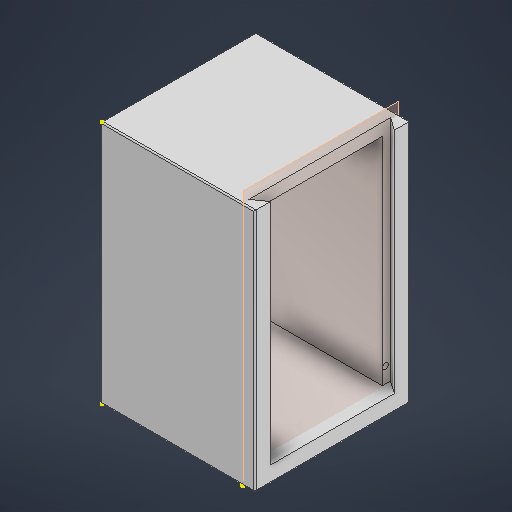
# Autodesk Inventor part: Part4
Saved by Autodesk Inventor 2026.1 (Build 301233000, 233)
## iProperties
Created: 2025-08-22
Part Number: Part4
Material: Generic
Document SubType Name: Modeling
Designer: usman
Density: 1 g/cm^3
Appearance: Default
Author: usman
Autodesk Inventor part; units mm, degrees
(part 1 of 2)
ref_plane "YZ Plane" through (0, 0, 0) normal (1, 0, 0) x (0, 1, 0)
ref_plane "XZ Plane" through (0, 0, 0) normal (0, 1, 0) x (-1, 0, 0)
ref_plane "XY Plane" through (0, 0, 0) normal (0, 0, 1) x (1, 0, 0)
sketch "Sketch1" plane through (0, 0, 0) normal (1, 0, 0) x (0, 1, 0)
  line L0 (0, 0) -> (191.4, 0)
  line L1 (191.4, 0) -> (191.4, -121.8)
  line L2 (191.4, -121.8) -> (0, -121.8)
  line L3 (0, -121.8) -> (0, 0)
  dimension "d0" = 191.4
  dimension "d1" = 121.8
  constraints: 8 end point, 2 parallel, 1 horizontal, 1 perpendicular
  measures "d0" distance of L0.start L0.end
  measures "d1" distance of L0.end L1.end
extrude "Extrusion1" add sketch "Sketch1" along normal blind 120
sketch "Sketch2" plane through (120, 0, 0) normal (1, 0, 0) x (0, 0, -1)
  line L0 (12.4, 178.9) -> (109.4, 178.9)
  line L1 (109.4, 178.9) -> (109.4, 12.5)
  line L2 (109.4, 12.5) -> (12.4, 12.5)
  line L3 (12.4, 12.5) -> (12.4, 178.9)
  line L4 (121.8, 191.4) -> (0, 191.4) projected
  line L5 (0, 0) -> (121.8, 0) projected
  line L6 (0, 191.4) -> (0, 0) projected
  dimension "d4" = 12.5
  dimension "d5" = 12.5
  dimension "d6" = 12.4
  dimension "d7" = 97
  constraints: 8 end point, 2 parallel, 1 horizontal, 1 perpendicular
  measures "d4" distance between parallel lines of L4 L0
  measures "d5" distance between parallel lines of L5 L2
  measures "d6" distance between parallel lines of L6 L3
  measures "d7" distance of L1.end L2.end
extrude "Extrusion2" cut sketch "Sketch2" against normal blind 105
sketch "Sketch3" plane through (0, 191.4, 0) normal (0, 1, 0) x (1, 0, 0)
  point P0 (0, 0)
sketch "Sketch4" plane through (0, 191.4, 0) normal (0, 1, 0) x (1, 0, 0)
  line L0 (120, 109.4) -> (15, 109.4) projected
  line L1 (120, 109.4) -> (110, 116.4021)
  line L2 (120, 121.8) -> (120, 0) projected
  line L3 (120, 60.9) -> (110, 60.9)
  line L4 (110, 60.9) -> (110, 116.4021)
  line L5 (120, 109.4) -> (120, 60.9)
  point P0 (0, 0)
  point P1 (106.1473, 60.9)
  dimension "d10" = 55
  dimension "d11" = 10
  constraints: 8 end point, 1 collinear, 1 horizontal, 1 midpoint, 1 perpendicular
  measures "d10" angle of L2 L1
  measures "d11" horizontal distance of L0.start L1.end
extrude "Extrusion3" cut sketch "Sketch4" against normal up to surface (178.9 mm away)
sketch "Sketch5" plane through (0, 191.4, 0) normal (0, 1, 0) x (1, 0, 0)
  line L0 (120, 109.4) -> (120, 12.4) projected
  line L1 (120, 12.4) -> (15, 12.4) projected
  line L2 (120, 60.9) -> (120, 12.4)
  line L3 (120, 12.4) -> (110, 5.3979)
  line L4 (120, 60.9) -> (120, 0) projected
  line L5 (110, 109.4) -> (110, 60.9) projected
  line L6 (110, 60.9) -> (110, 5.3979)
  line L7 (110, 60.9) -> (110, 5.3979)
  line L8 (110, 60.9) -> (120, 60.9) projected
  line L9 (120, 60.9) -> (110, 60.9)
  point P0 (0, 0)
  dimension "d14" = 10
  dimension "d15" = 125
  constraints: 10 end point, 2 collinear, 1 midpoint, 1 perpendicular, 1 vertical
  measures "d14" horizontal distance of L0.end L3.end
  measures "d15" angle of L4 L3
extrude "Extrusion4" cut sketch "Sketch5" against normal up to surface (178.9 mm away)
fillet "Fillet1" radius 1 7 edges at (60, 191.4, 0) (60, 0, 0) (60, 191.4, -121.8) (60, 0, -121.8) (120, 95.7, -121.8) (120, 0, -60.9) (120, 95.7, 0)
sketch "Sketch7" plane through (0, 0, -120.8) normal (0, -1, 0) x (1, 0, 0)
  point P0 (0, 120.8)
sketch "Sketch9" plane through (0, 0, -120.8) normal (0, -1, 0) x (1, 0, 0)
  line L0 (38.885, 112.5851) -> (86.602, 112.5851) construction
  line L1 (86.602, 112.5851) -> (86.602, 8.2699) construction
  line L2 (86.602, 8.2699) -> (38.885, 8.2699) construction
  line L3 (38.885, 8.2699) -> (38.885, 112.5851) construction
  line L4 (41.713, 65.0369) -> (41.7857, 63.9578)
  line L5 (41.7857, 63.9578) -> (41.713, 63.9578)
  spline S0 degree 2 poles (41.713, 63.9578) (41.5678, 64.4429) (41.0308, 64.8709) (40.6547, 64.8709) knots 0 0 0 1 2 2 2
  spline S1 degree 2 poles (40.6547, 64.8709) (40.3408, 64.8709) (39.8324, 64.5492) (39.5393, 63.8463) (39.5393, 63.3223) knots 0 0 0 1 2 3 3 3
  spline S2 degree 2 poles (39.5393, 63.3223) (39.5393, 62.8917) (39.8143, 62.2588) (40.3694, 61.9216) (40.7221, 61.9216) knots 0 0 0 1 2 3 3 3
  spline S3 degree 2 poles (40.7221, 61.9216) (41.0308, 61.9216) (41.5029, 62.1861) (41.7857, 62.5804) knots 0 0 0 1 2 2 2
  line L6 (41.7857, 62.5804) -> (41.8583, 62.5337)
  spline S4 degree 2 poles (41.8583, 62.5337) (41.6196, 62.1109) (40.9841, 61.7166) (40.5457, 61.7166) knots 0 0 0 1 2 2 2
  spline S5 degree 2 poles (40.5457, 61.7166) (39.7572, 61.7166) (39.324, 62.3029) knots 0 0 0 1 1 1
  spline S6 degree 2 poles (39.324, 62.3029) (39.0023, 62.7387) (39.0023, 63.3275) knots 0 0 0 1 1 1
  spline S7 degree 2 poles (39.0023, 63.3275) (39.0023, 63.8022) (39.4278, 64.5985) (40.1748, 65.0369) (40.6158, 65.0369) knots 0 0 0 1 2 3 3 3
  spline S8 degree 2 poles (40.6158, 65.0369) (40.9582, 65.0369) (41.2928, 64.8683) knots 0 0 0 1 1 1
  spline S9 degree 2 poles (41.2928, 64.8683) (41.3914, 64.8164) (41.4329, 64.8164) knots 0 0 0 1 1 1
  spline S10 degree 2 poles (41.4329, 64.8164) (41.4977, 64.8164) (41.5444, 64.8605) knots 0 0 0 1 1 1
  spline S11 degree 2 poles (41.5444, 64.8605) (41.6041, 64.9254) (41.63, 65.0369) knots 0 0 0 1 1 1
  line L7 (41.63, 65.0369) -> (41.713, 65.0369)
  spline S12 degree 2 poles (43.3887, 62.1005) (43.0593, 61.8437) (42.9737, 61.8048) knots 0 0 0 1 1 1
  spline S13 degree 2 poles (42.9737, 61.8048) (42.8492, 61.7452) (42.7065, 61.7452) knots 0 0 0 1 1 1
  spline S14 degree 2 poles (42.7065, 61.7452) (42.4834, 61.7452) (42.1955, 62.0487) (42.1955, 62.2977) knots 0 0 0 1 2 2 2
  spline S15 degree 2 poles (42.1955, 62.2977) (42.1955, 62.4533) (42.2655, 62.5701) knots 0 0 0 1 1 1
  spline S16 degree 2 poles (42.2655, 62.5701) (42.3615, 62.7283) (42.8362, 63.0084) (43.3887, 63.2108) knots 0 0 0 1 2 2 2
  line L8 (43.3887, 63.2108) -> (43.3887, 63.2938)
  spline S17 degree 2 poles (43.3887, 63.2938) (43.3887, 63.6154) (43.1864, 63.8541) (42.9918, 63.8541) knots 0 0 0 1 2 2 2
  spline S18 degree 2 poles (42.9918, 63.8541) (42.8466, 63.8541) (42.7584, 63.7736) knots 0 0 0 1 1 1
  spline S19 degree 2 poles (42.7584, 63.7736) (42.6702, 63.6958) (42.6702, 63.5921) knots 0 0 0 1 1 1
  line L9 (42.6702, 63.5921) -> (42.6754, 63.4572)
  spline S20 degree 2 poles (42.6754, 63.4572) (42.6754, 63.3482) (42.5638, 63.2315) (42.4757, 63.2315) knots 0 0 0 1 2 2 2
  spline S21 degree 2 poles (42.4757, 63.2315) (42.39, 63.2315) (42.2785, 63.3534) (42.2785, 63.4598) knots 0 0 0 1 2 2 2
  spline S22 degree 2 poles (42.2785, 63.4598) (42.2785, 63.6595) (42.6909, 63.9967) (43.0619, 63.9967) knots 0 0 0 1 2 2 2
  spline S23 degree 2 poles (43.0619, 63.9967) (43.3472, 63.9967) (43.5288, 63.9008) knots 0 0 0 1 1 1
  spline S24 degree 2 poles (43.5288, 63.9008) (43.6689, 63.8281) (43.7337, 63.6751) knots 0 0 0 1 1 1
  spline S25 degree 2 poles (43.7337, 63.6751) (43.7752, 63.5739) (43.7752, 63.2626) knots 0 0 0 1 1 1
  line L10 (43.7752, 63.2626) -> (43.7752, 62.5337)
  spline S26 degree 2 poles (43.7752, 62.5337) (43.7752, 62.2277) (43.7986, 62.0902) (43.853, 62.0435) (43.8868, 62.0435) knots 0 0 0 1 2 3 3 3
  spline S27 degree 2 poles (43.8868, 62.0435) (43.9257, 62.0435) (43.9542, 62.059) knots 0 0 0 1 1 1
  spline S28 degree 2 poles (43.9542, 62.059) (44.0035, 62.0902) (44.1436, 62.2302) knots 0 0 0 1 1 1
  line L11 (44.1436, 62.2302) -> (44.1436, 62.1005)
  spline S29 degree 2 poles (44.1436, 62.1005) (43.8816, 61.7478) (43.6429, 61.7478) knots 0 0 0 1 1 1
  spline S30 degree 2 poles (43.6429, 61.7478) (43.5262, 61.7478) (43.3913, 61.906) (43.3887, 62.1005) knots 0 0 0 1 2 2 2
  line L12 (43.3887, 62.251) -> (43.3887, 63.0681)
  spline S31 degree 2 poles (43.3887, 63.0681) (43.0359, 62.928) (42.9322, 62.8684) knots 0 0 0 1 1 1
  spline S32 degree 2 poles (42.9322, 62.8684) (42.748, 62.7672) (42.5898, 62.5415) (42.5898, 62.4092) knots 0 0 0 1 2 2 2
  spline S33 degree 2 poles (42.5898, 62.4092) (42.5898, 62.2406) (42.7895, 62.0175) (42.9218, 62.0175) knots 0 0 0 1 2 2 2
  spline S34 degree 2 poles (42.9218, 62.0175) (43.0982, 62.0175) (43.3887, 62.251) knots 0 0 0 1 1 1
  line L13 (45.6896, 63.9967) -> (45.6896, 63.2652)
  line L14 (45.6896, 63.2652) -> (45.6117, 63.2652)
  spline S35 degree 2 poles (45.6117, 63.2652) (45.5235, 63.6102) (45.246, 63.8592) (45.0307, 63.8592) knots 0 0 0 1 2 2 2
  spline S36 degree 2 poles (45.0307, 63.8592) (44.8673, 63.8592) (44.6649, 63.6855) (44.6649, 63.5817) knots 0 0 0 1 2 2 2
  spline S37 degree 2 poles (44.6649, 63.5817) (44.6649, 63.4494) (44.7402, 63.356) knots 0 0 0 1 1 1
  spline S38 degree 2 poles (44.7402, 63.356) (44.8102, 63.26) (45.0333, 63.1511) knots 0 0 0 1 1 1
  line L15 (45.0333, 63.1511) -> (45.3757, 62.9851)
  spline S39 degree 2 poles (45.3757, 62.9851) (45.8504, 62.7542) (45.8504, 62.3755) knots 0 0 0 1 1 1
  spline S40 degree 2 poles (45.8504, 62.3755) (45.8504, 62.0824) (45.4094, 61.7244) (45.1345, 61.7244) knots 0 0 0 1 2 2 2
  spline S41 degree 2 poles (45.1345, 61.7244) (44.9373, 61.7244) (44.6857, 61.7945) knots 0 0 0 1 1 1
  spline S42 degree 2 poles (44.6857, 61.7945) (44.6079, 61.8178) (44.5586, 61.8178) knots 0 0 0 1 1 1
  spline S43 degree 2 poles (44.5586, 61.8178) (44.5067, 61.8178) (44.4756, 61.7581) knots 0 0 0 1 1 1
  line L16 (44.4756, 61.7581) -> (44.3978, 61.7581)
  line L17 (44.3978, 61.7581) -> (44.3978, 62.5234)
  line L18 (44.3978, 62.5234) -> (44.4756, 62.5234)
  spline S44 degree 2 poles (44.4756, 62.5234) (44.5404, 62.1939) (44.9088, 61.8619) (45.1396, 61.8619) knots 0 0 0 1 2 2 2
  spline S45 degree 2 poles (45.1396, 61.8619) (45.3005, 61.8619) (45.5028, 62.0513) (45.5028, 62.1861) knots 0 0 0 1 2 2 2
  spline S46 degree 2 poles (45.5028, 62.1861) (45.5028, 62.347) (45.2771, 62.5675) (44.5975, 62.9021) (44.4912, 63.0396) knots 0 0 0 1 2 3 3 3
  spline S47 degree 2 poles (44.4912, 63.0396) (44.3874, 63.1718) (44.3874, 63.3768) knots 0 0 0 1 1 1
  spline S48 degree 2 poles (44.3874, 63.3768) (44.3874, 63.6414) (44.7505, 63.9967) (45.0385, 63.9967) knots 0 0 0 1 2 2 2
  spline S49 degree 2 poles (45.0385, 63.9967) (45.1656, 63.9967) (45.3446, 63.9423) knots 0 0 0 1 1 1
  spline S50 degree 2 poles (45.3446, 63.9423) (45.4639, 63.9085) (45.5028, 63.9085) knots 0 0 0 1 1 1
  spline S51 degree 2 poles (45.5028, 63.9085) (45.5417, 63.9085) (45.5832, 63.9423) (45.6117, 63.9967) knots 0 0 0 1 2 2 2
  line L19 (45.6117, 63.9967) -> (45.6896, 63.9967)
  line L20 (46.9113, 63.9967) -> (46.9113, 62.2743)
  spline S52 degree 2 poles (46.9113, 62.2743) (46.9113, 62.0746) (46.9684, 61.9397) (47.0851, 61.8749) (47.2356, 61.8749) knots 0 0 0 1 2 3 3 3
  line L21 (47.2356, 61.8749) -> (47.2356, 61.7893)
  line L22 (47.2356, 61.7893) -> (46.1954, 61.7893)
  line L23 (46.1954, 61.7893) -> (46.1954, 61.8749)
  spline S53 degree 2 poles (46.1954, 61.8749) (46.351, 61.8749) (46.46, 61.9345) (46.5222, 62.0746) (46.5222, 62.2743) knots 0 0 0 1 2 3 3 3
  line L24 (46.5222, 62.2743) -> (46.5222, 63.0992)
  spline S54 degree 2 poles (46.5222, 63.0992) (46.5222, 63.4468) (46.5015, 63.5506) knots 0 0 0 1 1 1
  spline S55 degree 2 poles (46.5015, 63.5506) (46.4859, 63.6258) (46.4133, 63.6855) (46.3536, 63.6855) knots 0 0 0 1 2 2 2
  spline S56 degree 2 poles (46.3536, 63.6855) (46.2888, 63.6855) (46.1954, 63.6491) knots 0 0 0 1 1 1
  line L25 (46.1954, 63.6491) -> (46.1617, 63.7347)
  line L26 (46.1617, 63.7347) -> (46.8076, 63.9967)
  line L27 (46.8076, 63.9967) -> (46.9113, 63.9967)
  spline S57 degree 2 poles (46.7168, 65.1199) (46.8153, 65.1199) (46.9528, 64.9824) (46.9528, 64.8839) knots 0 0 0 1 2 2 2
  spline S58 degree 2 poles (46.9528, 64.8839) (46.9528, 64.7853) (46.8153, 64.6452) (46.7168, 64.6452) knots 0 0 0 1 2 2 2
  spline S59 degree 2 poles (46.7168, 64.6452) (46.6182, 64.6452) (46.4781, 64.7853) (46.4781, 64.8839) knots 0 0 0 1 2 2 2
  spline S60 degree 2 poles (46.4781, 64.8839) (46.4781, 64.9824) (46.6156, 65.1199) (46.7168, 65.1199) knots 0 0 0 1 2 2 2
  spline S61 degree 2 poles (48.1331, 63.5428) (48.5092, 63.9967) (48.8516, 63.9967) knots 0 0 0 1 1 1
  spline S62 degree 2 poles (48.8516, 63.9967) (49.0254, 63.9967) (49.277, 63.8203) (49.3522, 63.6206) knots 0 0 0 1 2 2 2
  spline S63 degree 2 poles (49.3522, 63.6206) (49.4041, 63.4805) (49.4041, 63.19) knots 0 0 0 1 1 1
  line L28 (49.4041, 63.19) -> (49.4041, 62.2743)
  spline S64 degree 2 poles (49.4041, 62.2743) (49.4041, 62.072) (49.4378, 61.9994) knots 0 0 0 1 1 1
  spline S65 degree 2 poles (49.4378, 61.9994) (49.4638, 61.9397) (49.5779, 61.8749) (49.7309, 61.8749) knots 0 0 0 1 2 2 2
  line L29 (49.7309, 61.8749) -> (49.7309, 61.7893)
  line L30 (49.7309, 61.7893) -> (48.6674, 61.7893)
  line L31 (48.6674, 61.7893) -> (48.6674, 61.8749)
  line L32 (48.6674, 61.8749) -> (48.7115, 61.8749)
  spline S66 degree 2 poles (48.7115, 61.8749) (48.862, 61.8749) (48.9813, 61.9657) (49.0046, 62.0539) knots 0 0 0 1 2 2 2
  spline S67 degree 2 poles (49.0046, 62.0539) (49.015, 62.0902) (49.015, 62.2743) knots 0 0 0 1 1 1
  line L33 (49.015, 62.2743) -> (49.015, 63.1511)
  spline S68 degree 2 poles (49.015, 63.1511) (49.015, 63.4442) (48.8646, 63.7088) (48.6856, 63.7088) knots 0 0 0 1 2 2 2
  spline S69 degree 2 poles (48.6856, 63.7088) (48.408, 63.7088) (48.1331, 63.4053) knots 0 0 0 1 1 1
  line L34 (48.1331, 63.4053) -> (48.1331, 62.2743)
  spline S70 degree 2 poles (48.1331, 62.2743) (48.1331, 62.0564) (48.159, 62.0046) knots 0 0 0 1 1 1
  spline S71 degree 2 poles (48.159, 62.0046) (48.1927, 61.9371) (48.3069, 61.8749) (48.4832, 61.8749) knots 0 0 0 1 2 2 2
  line L35 (48.4832, 61.8749) -> (48.4832, 61.7893)
  line L36 (48.4832, 61.7893) -> (47.4171, 61.7893)
  line L37 (47.4171, 61.7893) -> (47.4171, 61.8749)
  line L38 (47.4171, 61.8749) -> (47.4638, 61.8749)
  spline S72 degree 2 poles (47.4638, 61.8749) (47.6298, 61.8749) (47.744, 62.0409) (47.744, 62.2743) knots 0 0 0 1 2 2 2
  line L39 (47.744, 62.2743) -> (47.744, 63.0707)
  spline S73 degree 2 poles (47.744, 63.0707) (47.744, 63.4546) (47.7077, 63.6232) (47.635, 63.6855) (47.5754, 63.6855) knots 0 0 0 1 2 3 3 3
  spline S74 degree 2 poles (47.5754, 63.6855) (47.5105, 63.6855) (47.4197, 63.6491) knots 0 0 0 1 1 1
  line L40 (47.4197, 63.6491) -> (47.3834, 63.7347)
  line L41 (47.3834, 63.7347) -> (48.0319, 63.9967)
  line L42 (48.0319, 63.9967) -> (48.1331, 63.9967)
  line L43 (48.1331, 63.9967) -> (48.1331, 63.5428)
  spline S75 degree 2 poles (50.478, 62.5726) (50.2809, 62.6686) (50.0707, 63.011) (50.0707, 63.2211) knots 0 0 0 1 2 2 2
  spline S76 degree 2 poles (50.0707, 63.2211) (50.0707, 63.5376) (50.5506, 63.9967) (50.9268, 63.9967) knots 0 0 0 1 2 2 2
  spline S77 degree 2 poles (50.9268, 63.9967) (51.2328, 63.9967) (51.4585, 63.8463) knots 0 0 0 1 1 1
  line L44 (51.4585, 63.8463) -> (51.9125, 63.8463)
  spline S78 degree 2 poles (51.9125, 63.8463) (52.0136, 63.8463) (52.0473, 63.8359) (52.0551, 63.8203) knots 0 0 0 1 2 2 2
  spline S79 degree 2 poles (52.0551, 63.8203) (52.0681, 63.7996) (52.0681, 63.7451) knots 0 0 0 1 1 1
  spline S80 degree 2 poles (52.0681, 63.7451) (52.0681, 63.6855) (52.0551, 63.6621) knots 0 0 0 1 1 1
  spline S81 degree 2 poles (52.0551, 63.6621) (52.0499, 63.6491) (52.0136, 63.6362) (51.9125, 63.6362) knots 0 0 0 1 2 2 2
  line L45 (51.9125, 63.6362) -> (51.6323, 63.6362)
  spline S82 degree 2 poles (51.6323, 63.6362) (51.7646, 63.4676) (51.7646, 63.2056) knots 0 0 0 1 1 1
  spline S83 degree 2 poles (51.7646, 63.2056) (51.7646, 62.9047) (51.3055, 62.4793) (50.919, 62.4793) knots 0 0 0 1 2 2 2
  spline S84 degree 2 poles (50.919, 62.4793) (50.7607, 62.4793) (50.5921, 62.526) knots 0 0 0 1 1 1
  spline S85 degree 2 poles (50.5921, 62.526) (50.491, 62.4378) (50.4183, 62.3055) (50.4183, 62.2588) knots 0 0 0 1 2 2 2
  spline S86 degree 2 poles (50.4183, 62.2588) (50.4183, 62.2173) (50.4962, 62.142) (50.6077, 62.1265) knots 0 0 0 1 2 2 2
  spline S87 degree 2 poles (50.6077, 62.1265) (50.6725, 62.1161) (50.9371, 62.1109) knots 0 0 0 1 1 1
  spline S88 degree 2 poles (50.9371, 62.1109) (51.4196, 62.098) (51.5623, 62.0772) knots 0 0 0 1 1 1
  spline S89 degree 2 poles (51.5623, 62.0772) (51.7802, 62.0461) (52.0396, 61.7841) (52.0396, 61.5947) knots 0 0 0 1 2 2 2
  spline S90 degree 2 poles (52.0396, 61.5947) (52.0396, 61.3301) (51.7905, 61.0993) knots 0 0 0 1 1 1
  spline S91 degree 2 poles (51.7905, 61.0993) (51.4248, 60.7569) (50.836, 60.7569) knots 0 0 0 1 1 1
  spline S92 degree 2 poles (50.836, 60.7569) (50.3846, 60.7569) (50.0733, 60.9592) knots 0 0 0 1 1 1
  spline S93 degree 2 poles (50.0733, 60.9592) (49.897, 61.0759) (49.897, 61.203) knots 0 0 0 1 1 1
  spline S94 degree 2 poles (49.897, 61.203) (49.897, 61.2601) (49.9229, 61.3146) knots 0 0 0 1 1 1
  spline S95 degree 2 poles (49.9229, 61.3146) (49.9618, 61.4028) (50.0863, 61.5558) knots 0 0 0 1 1 1
  spline S96 degree 2 poles (50.0863, 61.5558) (50.1045, 61.5766) (50.325, 61.8074) knots 0 0 0 1 1 1
  spline S97 degree 2 poles (50.325, 61.8074) (50.2056, 61.8801) (50.1045, 61.9968) (50.1045, 62.0694) knots 0 0 0 1 2 2 2
  spline S98 degree 2 poles (50.1045, 62.0694) (50.1045, 62.1498) (50.2368, 62.3703) (50.478, 62.5726) knots 0 0 0 1 2 2 2
  spline S99 degree 2 poles (50.4547, 61.7893) (50.3431, 61.67) (50.2316, 61.465) (50.2316, 61.3794) knots 0 0 0 1 2 2 2
  spline S100 degree 2 poles (50.2316, 61.3794) (50.2316, 61.2679) (50.3665, 61.1849) knots 0 0 0 1 1 1
  spline S101 degree 2 poles (50.3665, 61.1849) (50.6025, 61.0396) (51.0461, 61.0396) knots 0 0 0 1 1 1
  spline S102 degree 2 poles (51.0461, 61.0396) (51.4663, 61.0396) (51.8684, 61.3353) (51.8684, 61.5013) knots 0 0 0 1 2 2 2
  spline S103 degree 2 poles (51.8684, 61.5013) (51.8684, 61.6233) (51.749, 61.6751) knots 0 0 0 1 1 1
  spline S104 degree 2 poles (51.749, 61.6751) (51.6271, 61.7244) (51.2666, 61.7348) knots 0 0 0 1 1 1
  spline S105 degree 2 poles (51.2666, 61.7348) (50.7374, 61.7478) (50.4547, 61.7893) knots 0 0 0 1 1 1
  spline S106 degree 2 poles (50.8852, 63.8852) (50.7115, 63.8852) (50.478, 63.6102) (50.478, 63.3249) knots 0 0 0 1 2 2 2
  spline S107 degree 2 poles (50.478, 63.3249) (50.478, 62.954) (50.6362, 62.7516) knots 0 0 0 1 1 1
  spline S108 degree 2 poles (50.6362, 62.7516) (50.7581, 62.596) (50.9475, 62.596) knots 0 0 0 1 1 1
  spline S109 degree 2 poles (50.9475, 62.596) (51.1239, 62.596) (51.3548, 62.8632) (51.3548, 63.1485) knots 0 0 0 1 2 2 2
  spline S110 degree 2 poles (51.3548, 63.1485) (51.3548, 63.5194) (51.1939, 63.7295) knots 0 0 0 1 1 1
  spline S111 degree 2 poles (51.1939, 63.7295) (51.0746, 63.8852) (50.8852, 63.8852) knots 0 0 0 1 1 1
  line L46 (54.343, 63.7659) -> (54.343, 62.3548)
  spline S112 degree 2 poles (54.343, 62.3548) (54.343, 62.0564) (54.4078, 61.9786) knots 0 0 0 1 1 1
  spline S113 degree 2 poles (54.4078, 61.9786) (54.496, 61.8749) (54.6413, 61.8749) knots 0 0 0 1 1 1
  line L47 (54.6413, 61.8749) -> (54.8358, 61.8749)
  line L48 (54.8358, 61.8749) -> (54.8358, 61.7893)
  line L49 (54.8358, 61.7893) -> (53.5518, 61.7893)
  line L50 (53.5518, 61.7893) -> (53.5518, 61.8749)
  line L51 (53.5518, 61.8749) -> (53.6478, 61.8749)
  spline S114 degree 2 poles (53.6478, 61.8749) (53.7412, 61.8749) (53.8942, 61.9683) (53.9539, 62.1265) (53.9539, 62.3548) knots 0 0 0 1 2 3 3 3
  line L52 (53.9539, 62.3548) -> (53.9539, 63.7659)
  line L53 (53.9539, 63.7659) -> (53.5363, 63.7659)
  line L54 (53.5363, 63.7659) -> (53.5363, 63.9345)
  line L55 (53.5363, 63.9345) -> (53.9539, 63.9345)
  line L56 (53.9539, 63.9345) -> (53.9539, 64.0745)
  spline S115 degree 2 poles (53.9539, 64.0745) (53.9539, 64.3962) (54.1614, 64.8398) (54.5868, 65.1147) (54.8514, 65.1147) knots 0 0 0 1 2 3 3 3
  spline S116 degree 2 poles (54.8514, 65.1147) (55.0978, 65.1147) (55.3053, 64.9565) knots 0 0 0 1 1 1
  spline S117 degree 2 poles (55.3053, 64.9565) (55.4402, 64.8501) (55.4402, 64.7204) knots 0 0 0 1 1 1
  spline S118 degree 2 poles (55.4402, 64.7204) (55.4402, 64.6504) (55.3183, 64.5259) (55.2483, 64.5259) knots 0 0 0 1 2 2 2
  spline S119 degree 2 poles (55.2483, 64.5259) (55.1938, 64.5259) (55.0745, 64.6037) (54.9007, 64.8579) (54.8281, 64.902) knots 0 0 0 1 2 3 3 3
  spline S120 degree 2 poles (54.8281, 64.902) (54.7554, 64.9461) (54.6672, 64.9461) knots 0 0 0 1 1 1
  spline S121 degree 2 poles (54.6672, 64.9461) (54.5583, 64.9461) (54.4078, 64.832) (54.343, 64.5907) (54.343, 64.0901) knots 0 0 0 1 2 3 3 3
  line L57 (54.343, 64.0901) -> (54.343, 63.9345)
  line L58 (54.343, 63.9345) -> (54.8955, 63.9345)
  line L59 (54.8955, 63.9345) -> (54.8955, 63.7659)
  line L60 (54.8955, 63.7659) -> (54.343, 63.7659)
  spline S122 degree 2 poles (56.1484, 63.9967) (56.636, 63.9967) (56.9292, 63.6258) knots 0 0 0 1 1 1
  spline S123 degree 2 poles (56.9292, 63.6258) (57.1808, 63.3119) (57.1808, 62.9021) knots 0 0 0 1 1 1
  spline S124 degree 2 poles (57.1808, 62.9021) (57.1808, 62.6141) (56.9032, 62.0227) (56.4207, 61.7244) (56.1224, 61.7244) knots 0 0 0 1 2 3 3 3
  spline S125 degree 2 poles (56.1224, 61.7244) (55.6374, 61.7244) (55.352, 62.1109) knots 0 0 0 1 1 1
  spline S126 degree 2 poles (55.352, 62.1109) (55.1108, 62.4352) (55.1108, 62.8398) knots 0 0 0 1 1 1
  spline S127 degree 2 poles (55.1108, 62.8398) (55.1108, 63.1355) (55.4039, 63.7192) (55.8812, 63.9967) (56.1484, 63.9967) knots 0 0 0 1 2 3 3 3
  spline S128 degree 2 poles (56.0758, 63.8437) (55.9512, 63.8437) (55.7022, 63.6958) (55.5466, 63.3275) (55.5466, 63.037) knots 0 0 0 1 2 3 3 3
  spline S129 degree 2 poles (55.5466, 63.037) (55.5466, 62.5701) (55.9175, 61.8904) (56.2236, 61.8904) knots 0 0 0 1 2 2 2
  spline S130 degree 2 poles (56.2236, 61.8904) (56.4493, 61.8904) (56.745, 62.264) (56.745, 62.7205) knots 0 0 0 1 2 2 2
  spline S131 degree 2 poles (56.745, 62.7205) (56.745, 63.2912) (56.4986, 63.618) knots 0 0 0 1 1 1
  spline S132 degree 2 poles (56.4986, 63.618) (56.3326, 63.8437) (56.0758, 63.8437) knots 0 0 0 1 1 1
  line L61 (58.1302, 63.9967) -> (58.1302, 63.5143)
  spline S133 degree 2 poles (58.1302, 63.5143) (58.3999, 63.9967) (58.6827, 63.9967) knots 0 0 0 1 1 1
  spline S134 degree 2 poles (58.6827, 63.9967) (58.8098, 63.9967) (58.9784, 63.8411) (58.9784, 63.7373) knots 0 0 0 1 2 2 2
  spline S135 degree 2 poles (58.9784, 63.7373) (58.9784, 63.6465) (58.8565, 63.5194) (58.7735, 63.5194) knots 0 0 0 1 2 2 2
  spline S136 degree 2 poles (58.7735, 63.5194) (58.6905, 63.5194) (58.4881, 63.6803) (58.4388, 63.6803) knots 0 0 0 1 2 2 2
  spline S137 degree 2 poles (58.4388, 63.6803) (58.3973, 63.6803) (58.3481, 63.6336) knots 0 0 0 1 1 1
  spline S138 degree 2 poles (58.3481, 63.6336) (58.2417, 63.5376) (58.1302, 63.3171) knots 0 0 0 1 1 1
  line L62 (58.1302, 63.3171) -> (58.1302, 62.2899)
  spline S139 degree 2 poles (58.1302, 62.2899) (58.1302, 62.1109) (58.1743, 62.0201) knots 0 0 0 1 1 1
  spline S140 degree 2 poles (58.1743, 62.0201) (58.2054, 61.9579) (58.3584, 61.8749) (58.5037, 61.8749) knots 0 0 0 1 2 2 2
  line L63 (58.5037, 61.8749) -> (58.5037, 61.7893)
  line L64 (58.5037, 61.7893) -> (57.4039, 61.7893)
  line L65 (57.4039, 61.7893) -> (57.4039, 61.8749)
  spline S141 degree 2 poles (57.4039, 61.8749) (57.5673, 61.8749) (57.6477, 61.9268) knots 0 0 0 1 1 1
  spline S142 degree 2 poles (57.6477, 61.9268) (57.7048, 61.9631) (57.7281, 62.0461) knots 0 0 0 1 1 1
  spline S143 degree 2 poles (57.7281, 62.0461) (57.7411, 62.0876) (57.7411, 62.2743) knots 0 0 0 1 1 1
  line L66 (57.7411, 62.2743) -> (57.7411, 63.1018)
  spline S144 degree 2 poles (57.7411, 63.1018) (57.7411, 63.4753) (57.7099, 63.618) (57.6295, 63.6855) (57.5673, 63.6855) knots 0 0 0 1 2 3 3 3
  spline S145 degree 2 poles (57.5673, 63.6855) (57.4946, 63.6855) (57.4039, 63.6491) knots 0 0 0 1 1 1
  line L67 (57.4039, 63.6491) -> (57.3805, 63.7347)
  line L68 (57.3805, 63.7347) -> (58.0316, 63.9967)
  line L69 (58.0316, 63.9967) -> (58.1302, 63.9967)
  line L70 (62.1093, 61.7893) -> (60.8798, 64.461)
  line L71 (60.8798, 64.461) -> (60.8798, 62.3392)
  spline S146 degree 2 poles (60.8798, 62.3392) (60.8798, 62.0461) (60.942, 61.9734) knots 0 0 0 1 1 1
  spline S147 degree 2 poles (60.942, 61.9734) (61.0302, 61.8749) (61.217, 61.8749) knots 0 0 0 1 1 1
  line L72 (61.217, 61.8749) -> (61.3285, 61.8749)
  line L73 (61.3285, 61.8749) -> (61.3285, 61.7893)
  line L74 (61.3285, 61.7893) -> (60.2261, 61.7893)
  line L75 (60.2261, 61.7893) -> (60.2261, 61.8749)
  line L76 (60.2261, 61.8749) -> (60.3376, 61.8749)
  spline S148 degree 2 poles (60.3376, 61.8749) (60.5399, 61.8749) (60.623, 61.9968) knots 0 0 0 1 1 1
  spline S149 degree 2 poles (60.623, 61.9968) (60.6748, 62.072) (60.6748, 62.3392) knots 0 0 0 1 1 1
  line L77 (60.6748, 62.3392) -> (60.6748, 64.4144)
  spline S150 degree 2 poles (60.6748, 64.4144) (60.6748, 64.6245) (60.6281, 64.7204) knots 0 0 0 1 1 1
  spline S151 degree 2 poles (60.6281, 64.7204) (60.5944, 64.7879) (60.4206, 64.8787) (60.2261, 64.8787) knots 0 0 0 1 2 2 2
  line L78 (60.2261, 64.8787) -> (60.2261, 64.9643)
  line L79 (60.2261, 64.9643) -> (61.1262, 64.9643)
  line L80 (61.1262, 64.9643) -> (62.2779, 62.4793)
  line L81 (62.2779, 62.4793) -> (63.414, 64.9643)
  line L82 (63.414, 64.9643) -> (64.309, 64.9643)
  line L83 (64.309, 64.9643) -> (64.309, 64.8787)
  line L84 (64.309, 64.8787) -> (64.2, 64.8787)
  spline S152 degree 2 poles (64.2, 64.8787) (63.9951, 64.8787) (63.9121, 64.7568) knots 0 0 0 1 1 1
  spline S153 degree 2 poles (63.9121, 64.7568) (63.8602, 64.6815) (63.8602, 64.4144) knots 0 0 0 1 1 1
  line L85 (63.8602, 64.4144) -> (63.8602, 62.3392)
  spline S154 degree 2 poles (63.8602, 62.3392) (63.8602, 62.0461) (63.9251, 61.9734) knots 0 0 0 1 1 1
  spline S155 degree 2 poles (63.9251, 61.9734) (64.0133, 61.8749) (64.2, 61.8749) knots 0 0 0 1 1 1
  line L86 (64.2, 61.8749) -> (64.309, 61.8749)
  line L87 (64.309, 61.8749) -> (64.309, 61.7893)
  line L88 (64.309, 61.7893) -> (62.9627, 61.7893)
  line L89 (62.9627, 61.7893) -> (62.9627, 61.8749)
  line L90 (62.9627, 61.8749) -> (63.0742, 61.8749)
  spline S156 degree 2 poles (63.0742, 61.8749) (63.2792, 61.8749) (63.3596, 61.9968) knots 0 0 0 1 1 1
  spline S157 degree 2 poles (63.3596, 61.9968) (63.4115, 62.072) (63.4115, 62.3392) knots 0 0 0 1 1 1
  line L91 (63.4115, 62.3392) -> (63.4115, 64.461)
  line L92 (63.4115, 64.461) -> (62.1871, 61.7893)
  line L93 (62.1871, 61.7893) -> (62.1093, 61.7893)
  spline S158 degree 2 poles (65.7745, 62.1005) (65.4451, 61.8437) (65.3595, 61.8048) knots 0 0 0 1 1 1
  spline S159 degree 2 poles (65.3595, 61.8048) (65.235, 61.7452) (65.0923, 61.7452) knots 0 0 0 1 1 1
  spline S160 degree 2 poles (65.0923, 61.7452) (64.8693, 61.7452) (64.5813, 62.0487) (64.5813, 62.2977) knots 0 0 0 1 2 2 2
  spline S161 degree 2 poles (64.5813, 62.2977) (64.5813, 62.4533) (64.6514, 62.5701) knots 0 0 0 1 1 1
  spline S162 degree 2 poles (64.6514, 62.5701) (64.7473, 62.7283) (65.222, 63.0084) (65.7745, 63.2108) knots 0 0 0 1 2 2 2
  line L94 (65.7745, 63.2108) -> (65.7745, 63.2938)
  spline S163 degree 2 poles (65.7745, 63.2938) (65.7745, 63.6154) (65.5722, 63.8541) (65.3777, 63.8541) knots 0 0 0 1 2 2 2
  spline S164 degree 2 poles (65.3777, 63.8541) (65.2324, 63.8541) (65.1442, 63.7736) knots 0 0 0 1 1 1
  spline S165 degree 2 poles (65.1442, 63.7736) (65.056, 63.6958) (65.056, 63.5921) knots 0 0 0 1 1 1
  line L95 (65.056, 63.5921) -> (65.0612, 63.4572)
  spline S166 degree 2 poles (65.0612, 63.4572) (65.0612, 63.3482) (64.9497, 63.2315) (64.8615, 63.2315) knots 0 0 0 1 2 2 2
  spline S167 degree 2 poles (64.8615, 63.2315) (64.7759, 63.2315) (64.6643, 63.3534) (64.6643, 63.4598) knots 0 0 0 1 2 2 2
  spline S168 degree 2 poles (64.6643, 63.4598) (64.6643, 63.6595) (65.0768, 63.9967) (65.4477, 63.9967) knots 0 0 0 1 2 2 2
  spline S169 degree 2 poles (65.4477, 63.9967) (65.733, 63.9967) (65.9146, 63.9008) knots 0 0 0 1 1 1
  spline S170 degree 2 poles (65.9146, 63.9008) (66.0547, 63.8281) (66.1195, 63.6751) knots 0 0 0 1 1 1
  spline S171 degree 2 poles (66.1195, 63.6751) (66.161, 63.5739) (66.161, 63.2626) knots 0 0 0 1 1 1
  line L96 (66.161, 63.2626) -> (66.161, 62.5337)
  spline S172 degree 2 poles (66.161, 62.5337) (66.161, 62.2277) (66.1844, 62.0902) (66.2389, 62.0435) (66.2726, 62.0435) knots 0 0 0 1 2 3 3 3
  spline S173 degree 2 poles (66.2726, 62.0435) (66.3115, 62.0435) (66.34, 62.059) knots 0 0 0 1 1 1
  spline S174 degree 2 poles (66.34, 62.059) (66.3893, 62.0902) (66.5294, 62.2302) knots 0 0 0 1 1 1
  line L97 (66.5294, 62.2302) -> (66.5294, 62.1005)
  spline S175 degree 2 poles (66.5294, 62.1005) (66.2674, 61.7478) (66.0288, 61.7478) knots 0 0 0 1 1 1
  spline S176 degree 2 poles (66.0288, 61.7478) (65.912, 61.7478) (65.7771, 61.906) (65.7745, 62.1005) knots 0 0 0 1 2 2 2
  line L98 (65.7745, 62.251) -> (65.7745, 63.0681)
  spline S177 degree 2 poles (65.7745, 63.0681) (65.4218, 62.928) (65.318, 62.8684) knots 0 0 0 1 1 1
  spline S178 degree 2 poles (65.318, 62.8684) (65.1338, 62.7672) (64.9756, 62.5415) (64.9756, 62.4092) knots 0 0 0 1 2 2 2
  spline S179 degree 2 poles (64.9756, 62.4092) (64.9756, 62.2406) (65.1753, 62.0175) (65.3076, 62.0175) knots 0 0 0 1 2 2 2
  spline S180 degree 2 poles (65.3076, 62.0175) (65.484, 62.0175) (65.7745, 62.251) knots 0 0 0 1 1 1
  spline S181 degree 2 poles (67.2635, 62.5726) (67.0663, 62.6686) (66.8562, 63.011) (66.8562, 63.2211) knots 0 0 0 1 2 2 2
  spline S182 degree 2 poles (66.8562, 63.2211) (66.8562, 63.5376) (67.3361, 63.9967) (67.7122, 63.9967) knots 0 0 0 1 2 2 2
  spline S183 degree 2 poles (67.7122, 63.9967) (68.0183, 63.9967) (68.244, 63.8463) knots 0 0 0 1 1 1
  line L99 (68.244, 63.8463) -> (68.6979, 63.8463)
  spline S184 degree 2 poles (68.6979, 63.8463) (68.7991, 63.8463) (68.8328, 63.8359) (68.8406, 63.8203) knots 0 0 0 1 2 2 2
  spline S185 degree 2 poles (68.8406, 63.8203) (68.8536, 63.7996) (68.8536, 63.7451) knots 0 0 0 1 1 1
  spline S186 degree 2 poles (68.8536, 63.7451) (68.8536, 63.6855) (68.8406, 63.6621) knots 0 0 0 1 1 1
  spline S187 degree 2 poles (68.8406, 63.6621) (68.8354, 63.6491) (68.7991, 63.6362) (68.6979, 63.6362) knots 0 0 0 1 2 2 2
  line L100 (68.6979, 63.6362) -> (68.4178, 63.6362)
  spline S188 degree 2 poles (68.4178, 63.6362) (68.5501, 63.4676) (68.5501, 63.2056) knots 0 0 0 1 1 1
  spline S189 degree 2 poles (68.5501, 63.2056) (68.5501, 62.9047) (68.0909, 62.4793) (67.7044, 62.4793) knots 0 0 0 1 2 2 2
  spline S190 degree 2 poles (67.7044, 62.4793) (67.5462, 62.4793) (67.3776, 62.526) knots 0 0 0 1 1 1
  spline S191 degree 2 poles (67.3776, 62.526) (67.2764, 62.4378) (67.2038, 62.3055) (67.2038, 62.2588) knots 0 0 0 1 2 2 2
  spline S192 degree 2 poles (67.2038, 62.2588) (67.2038, 62.2173) (67.2816, 62.142) (67.3932, 62.1265) knots 0 0 0 1 2 2 2
  spline S193 degree 2 poles (67.3932, 62.1265) (67.458, 62.1161) (67.7226, 62.1109) knots 0 0 0 1 1 1
  spline S194 degree 2 poles (67.7226, 62.1109) (68.2051, 62.098) (68.3477, 62.0772) knots 0 0 0 1 1 1
  spline S195 degree 2 poles (68.3477, 62.0772) (68.5656, 62.0461) (68.825, 61.7841) (68.825, 61.5947) knots 0 0 0 1 2 2 2
  spline S196 degree 2 poles (68.825, 61.5947) (68.825, 61.3301) (68.576, 61.0993) knots 0 0 0 1 1 1
  spline S197 degree 2 poles (68.576, 61.0993) (68.2103, 60.7569) (67.6214, 60.7569) knots 0 0 0 1 1 1
  spline S198 degree 2 poles (67.6214, 60.7569) (67.1701, 60.7569) (66.8588, 60.9592) knots 0 0 0 1 1 1
  spline S199 degree 2 poles (66.8588, 60.9592) (66.6824, 61.0759) (66.6824, 61.203) knots 0 0 0 1 1 1
  spline S200 degree 2 poles (66.6824, 61.203) (66.6824, 61.2601) (66.7084, 61.3146) knots 0 0 0 1 1 1
  spline S201 degree 2 poles (66.7084, 61.3146) (66.7473, 61.4028) (66.8718, 61.5558) knots 0 0 0 1 1 1
  spline S202 degree 2 poles (66.8718, 61.5558) (66.8899, 61.5766) (67.1104, 61.8074) knots 0 0 0 1 1 1
  spline S203 degree 2 poles (67.1104, 61.8074) (66.9911, 61.8801) (66.8899, 61.9968) (66.8899, 62.0694) knots 0 0 0 1 2 2 2
  spline S204 degree 2 poles (66.8899, 62.0694) (66.8899, 62.1498) (67.0222, 62.3703) (67.2635, 62.5726) knots 0 0 0 1 2 2 2
  spline S205 degree 2 poles (67.2401, 61.7893) (67.1286, 61.67) (67.0171, 61.465) (67.0171, 61.3794) knots 0 0 0 1 2 2 2
  spline S206 degree 2 poles (67.0171, 61.3794) (67.0171, 61.2679) (67.1519, 61.1849) knots 0 0 0 1 1 1
  spline S207 degree 2 poles (67.1519, 61.1849) (67.388, 61.0396) (67.8316, 61.0396) knots 0 0 0 1 1 1
  spline S208 degree 2 poles (67.8316, 61.0396) (68.2518, 61.0396) (68.6538, 61.3353) (68.6538, 61.5013) knots 0 0 0 1 2 2 2
  spline S209 degree 2 poles (68.6538, 61.5013) (68.6538, 61.6233) (68.5345, 61.6751) knots 0 0 0 1 1 1
  spline S210 degree 2 poles (68.5345, 61.6751) (68.4126, 61.7244) (68.052, 61.7348) knots 0 0 0 1 1 1
  spline S211 degree 2 poles (68.052, 61.7348) (67.5229, 61.7478) (67.2401, 61.7893) knots 0 0 0 1 1 1
  spline S212 degree 2 poles (67.6707, 63.8852) (67.4969, 63.8852) (67.2635, 63.6102) (67.2635, 63.3249) knots 0 0 0 1 2 2 2
  spline S213 degree 2 poles (67.2635, 63.3249) (67.2635, 62.954) (67.4217, 62.7516) knots 0 0 0 1 1 1
  spline S214 degree 2 poles (67.4217, 62.7516) (67.5436, 62.596) (67.733, 62.596) knots 0 0 0 1 1 1
  spline S215 degree 2 poles (67.733, 62.596) (67.9094, 62.596) (68.1402, 62.8632) (68.1402, 63.1485) knots 0 0 0 1 2 2 2
  spline S216 degree 2 poles (68.1402, 63.1485) (68.1402, 63.5194) (67.9794, 63.7295) knots 0 0 0 1 1 1
  spline S217 degree 2 poles (67.9794, 63.7295) (67.8601, 63.8852) (67.6707, 63.8852) knots 0 0 0 1 1 1
  spline S218 degree 2 poles (69.7174, 63.5428) (70.0935, 63.9967) (70.4359, 63.9967) knots 0 0 0 1 1 1
  spline S219 degree 2 poles (70.4359, 63.9967) (70.6097, 63.9967) (70.8613, 63.8203) (70.9365, 63.6206) knots 0 0 0 1 2 2 2
  spline S220 degree 2 poles (70.9365, 63.6206) (70.9884, 63.4805) (70.9884, 63.19) knots 0 0 0 1 1 1
  line L101 (70.9884, 63.19) -> (70.9884, 62.2743)
  spline S221 degree 2 poles (70.9884, 62.2743) (70.9884, 62.072) (71.0221, 61.9994) knots 0 0 0 1 1 1
  spline S222 degree 2 poles (71.0221, 61.9994) (71.0481, 61.9397) (71.1622, 61.8749) (71.3152, 61.8749) knots 0 0 0 1 2 2 2
  line L102 (71.3152, 61.8749) -> (71.3152, 61.7893)
  line L103 (71.3152, 61.7893) -> (70.2517, 61.7893)
  line L104 (70.2517, 61.7893) -> (70.2517, 61.8749)
  line L105 (70.2517, 61.8749) -> (70.2958, 61.8749)
  spline S223 degree 2 poles (70.2958, 61.8749) (70.4463, 61.8749) (70.5656, 61.9657) (70.5889, 62.0539) knots 0 0 0 1 2 2 2
  spline S224 degree 2 poles (70.5889, 62.0539) (70.5993, 62.0902) (70.5993, 62.2743) knots 0 0 0 1 1 1
  line L106 (70.5993, 62.2743) -> (70.5993, 63.1511)
  spline S225 degree 2 poles (70.5993, 63.1511) (70.5993, 63.4442) (70.4489, 63.7088) (70.2699, 63.7088) knots 0 0 0 1 2 2 2
  spline S226 degree 2 poles (70.2699, 63.7088) (69.9923, 63.7088) (69.7174, 63.4053) knots 0 0 0 1 1 1
  line L107 (69.7174, 63.4053) -> (69.7174, 62.2743)
  spline S227 degree 2 poles (69.7174, 62.2743) (69.7174, 62.0564) (69.7433, 62.0046) knots 0 0 0 1 1 1
  spline S228 degree 2 poles (69.7433, 62.0046) (69.777, 61.9371) (69.8912, 61.8749) (70.0675, 61.8749) knots 0 0 0 1 2 2 2
  line L108 (70.0675, 61.8749) -> (70.0675, 61.7893)
  line L109 (70.0675, 61.7893) -> (69.0014, 61.7893)
  line L110 (69.0014, 61.7893) -> (69.0014, 61.8749)
  line L111 (69.0014, 61.8749) -> (69.0481, 61.8749)
  spline S229 degree 2 poles (69.0481, 61.8749) (69.2141, 61.8749) (69.3283, 62.0409) (69.3283, 62.2743) knots 0 0 0 1 2 2 2
  line L112 (69.3283, 62.2743) -> (69.3283, 63.0707)
  spline S230 degree 2 poles (69.3283, 63.0707) (69.3283, 63.4546) (69.2919, 63.6232) (69.2193, 63.6855) (69.1597, 63.6855) knots 0 0 0 1 2 3 3 3
  spline S231 degree 2 poles (69.1597, 63.6855) (69.0948, 63.6855) (69.004, 63.6491) knots 0 0 0 1 1 1
  line L113 (69.004, 63.6491) -> (68.9677, 63.7347)
  line L114 (68.9677, 63.7347) -> (69.6162, 63.9967)
  line L115 (69.6162, 63.9967) -> (69.7174, 63.9967)
  line L116 (69.7174, 63.9967) -> (69.7174, 63.5428)
  spline S232 degree 2 poles (71.8496, 63.1252) (71.847, 62.6479) (72.0804, 62.3781) knots 0 0 0 1 1 1
  spline S233 degree 2 poles (72.0804, 62.3781) (72.3165, 62.1057) (72.633, 62.1057) knots 0 0 0 1 1 1
  spline S234 degree 2 poles (72.633, 62.1057) (72.8431, 62.1057) (73.1543, 62.3366) (73.2607, 62.6193) knots 0 0 0 1 2 2 2
  line L117 (73.2607, 62.6193) -> (73.3333, 62.5726)
  spline S235 degree 2 poles (73.3333, 62.5726) (73.284, 62.251) (72.8119, 61.7244) (72.454, 61.7244) knots 0 0 0 1 2 2 2
  spline S236 degree 2 poles (72.454, 61.7244) (72.0675, 61.7244) (71.5176, 62.3262) (71.5176, 62.832) knots 0 0 0 1 2 2 2
  spline S237 degree 2 poles (71.5176, 62.832) (71.5176, 63.382) (72.083, 63.9967) (72.5085, 63.9967) knots 0 0 0 1 2 2 2
  spline S238 degree 2 poles (72.5085, 63.9967) (72.869, 63.9967) (73.3333, 63.522) (73.3333, 63.1252) knots 0 0 0 1 2 2 2
  line L118 (73.3333, 63.1252) -> (71.8496, 63.1252)
  line L119 (71.8496, 63.26) -> (72.8457, 63.26)
  spline S239 degree 2 poles (72.8457, 63.26) (72.8327, 63.465) (72.7964, 63.5506) knots 0 0 0 1 1 1
  spline S240 degree 2 poles (72.7964, 63.5506) (72.7367, 63.6803) (72.5059, 63.8307) (72.3788, 63.8307) knots 0 0 0 1 2 2 2
  spline S241 degree 2 poles (72.3788, 63.8307) (72.1842, 63.8307) (71.8755, 63.5298) (71.8496, 63.26) knots 0 0 0 1 2 2 2
  line L120 (74.2438, 64.64) -> (74.2438, 63.9345)
  line L121 (74.2438, 63.9345) -> (74.7444, 63.9345)
  line L122 (74.7444, 63.9345) -> (74.7444, 63.7711)
  line L123 (74.7444, 63.7711) -> (74.2438, 63.7711)
  line L124 (74.2438, 63.7711) -> (74.2438, 62.3781)
  spline S242 degree 2 poles (74.2438, 62.3781) (74.2438, 62.1706) (74.3631, 62.0253) (74.4565, 62.0253) knots 0 0 0 1 2 2 2
  spline S243 degree 2 poles (74.4565, 62.0253) (74.5343, 62.0253) (74.6822, 62.1213) (74.7211, 62.2147) knots 0 0 0 1 2 2 2
  line L125 (74.7211, 62.2147) -> (74.8119, 62.2147)
  spline S244 degree 2 poles (74.8119, 62.2147) (74.7289, 61.9838) (74.428, 61.753) (74.2697, 61.753) knots 0 0 0 1 2 2 2
  spline S245 degree 2 poles (74.2697, 61.753) (74.1608, 61.753) (73.9533, 61.8723) (73.8547, 62.0954) (73.8547, 62.3262) knots 0 0 0 1 2 3 3 3
  line L126 (73.8547, 62.3262) -> (73.8547, 63.7711)
  line L127 (73.8547, 63.7711) -> (73.5149, 63.7711)
  line L128 (73.5149, 63.7711) -> (73.5149, 63.8489)
  spline S246 degree 2 poles (73.5149, 63.8489) (73.6446, 63.9008) (73.9144, 64.1446) (74.0207, 64.3132) knots 0 0 0 1 2 2 2
  spline S247 degree 2 poles (74.0207, 64.3132) (74.0752, 64.404) (74.1712, 64.64) knots 0 0 0 1 1 1
  line L129 (74.1712, 64.64) -> (74.2438, 64.64)
  line L130 (78.1996, 62.8502) -> (76.9649, 62.8502)
  line L131 (76.9649, 62.8502) -> (76.7496, 62.3522)
  spline S248 degree 2 poles (76.7496, 62.3522) (76.6692, 62.1654) (76.6692, 62.0746) knots 0 0 0 1 1 1
  spline S249 degree 2 poles (76.6692, 62.0746) (76.6692, 62.002) (76.8092, 61.8904) (77.0375, 61.8749) knots 0 0 0 1 2 2 2
  line L132 (77.0375, 61.8749) -> (77.0375, 61.7893)
  line L133 (77.0375, 61.7893) -> (76.0362, 61.7893)
  line L134 (76.0362, 61.7893) -> (76.0362, 61.8749)
  spline S250 degree 2 poles (76.0362, 61.8749) (76.236, 61.9112) (76.293, 61.9657) knots 0 0 0 1 1 1
  spline S251 degree 2 poles (76.293, 61.9657) (76.4124, 62.0798) (76.5576, 62.4248) knots 0 0 0 1 1 1
  line L135 (76.5576, 62.4248) -> (77.6782, 65.0369)
  line L136 (77.6782, 65.0369) -> (77.7612, 65.0369)
  line L137 (77.7612, 65.0369) -> (78.8662, 62.3963)
  spline S252 degree 2 poles (78.8662, 62.3963) (78.9985, 62.0772) (79.2164, 61.8878) (79.411, 61.8749) knots 0 0 0 1 2 2 2
  line L138 (79.411, 61.8749) -> (79.411, 61.7893)
  line L139 (79.411, 61.7893) -> (78.1581, 61.7893)
  line L140 (78.1581, 61.7893) -> (78.1581, 61.8749)
  spline S253 degree 2 poles (78.1581, 61.8749) (78.3474, 61.8852) (78.4823, 61.9916) (78.4823, 62.0694) knots 0 0 0 1 2 2 2
  spline S254 degree 2 poles (78.4823, 62.0694) (78.4823, 62.1732) (78.3889, 62.3963) knots 0 0 0 1 1 1
  line L141 (78.3889, 62.3963) -> (78.1996, 62.8502)
  line L142 (78.127, 63.024) -> (77.5926, 64.308)
  line L143 (77.5926, 64.308) -> (77.0375, 63.024)
  line L144 (77.0375, 63.024) -> (78.127, 63.024)
  line L145 (81.6158, 65.0291) -> (81.6158, 64.9435)
  spline S255 degree 2 poles (81.6158, 64.9435) (81.3071, 64.9124) (80.9129, 64.7282) (80.5316, 64.3495) (80.2799, 63.8826) (80.1943, 63.5609) knots 0 0 0 1 2 3 4 4 4
  spline S256 degree 2 poles (80.1943, 63.5609) (80.5341, 63.7944) (80.874, 63.7944) knots 0 0 0 1 1 1
  spline S257 degree 2 poles (80.874, 63.7944) (81.1982, 63.7944) (81.6781, 63.2704) (81.6781, 62.858) knots 0 0 0 1 2 2 2
  spline S258 degree 2 poles (81.6781, 62.858) (81.6781, 62.4611) (81.4368, 62.1317) knots 0 0 0 1 1 1
  spline S259 degree 2 poles (81.4368, 62.1317) (81.1463, 61.7348) (80.6664, 61.7348) knots 0 0 0 1 1 1
  spline S260 degree 2 poles (80.6664, 61.7348) (80.3422, 61.7348) (80.1139, 61.9501) knots 0 0 0 1 1 1
  spline S261 degree 2 poles (80.1139, 61.9501) (79.6678, 62.3677) (79.6678, 63.037) knots 0 0 0 1 1 1
  spline S262 degree 2 poles (79.6678, 63.037) (79.6678, 63.4624) (80.0102, 64.2302) (80.6457, 64.8242) (81.2293, 65.0291) (81.4809, 65.0291) knots 0 0 0 1 2 3 4 4 4
  line L146 (81.4809, 65.0291) -> (81.6158, 65.0291)
  spline S263 degree 2 poles (80.1554, 63.3897) (80.1139, 63.0759) (80.1139, 62.8813) knots 0 0 0 1 1 1
  spline S264 degree 2 poles (80.1139, 62.8813) (80.1139, 62.6582) (80.2799, 62.1317) (80.4434, 61.976) knots 0 0 0 1 2 2 2
  spline S265 degree 2 poles (80.4434, 61.976) (80.5653, 61.8671) (80.7365, 61.8671) knots 0 0 0 1 1 1
  spline S266 degree 2 poles (80.7365, 61.8671) (80.9388, 61.8671) (81.2605, 62.251) (81.2605, 62.6064) knots 0 0 0 1 2 2 2
  spline S267 degree 2 poles (81.2605, 62.6064) (81.2605, 63.0058) (80.9414, 63.5895) (80.6483, 63.5895) knots 0 0 0 1 2 2 2
  spline S268 degree 2 poles (80.6483, 63.5895) (80.5601, 63.5895) (80.3552, 63.5143) (80.1554, 63.3897) knots 0 0 0 1 2 2 2
  line L147 (84.0956, 62.9591) -> (84.0956, 62.6271)
  line L148 (84.0956, 62.6271) -> (83.6702, 62.6271)
  line L149 (83.6702, 62.6271) -> (83.6702, 61.7893)
  line L150 (83.6702, 61.7893) -> (83.2837, 61.7893)
  line L151 (83.2837, 61.7893) -> (83.2837, 62.6271)
  line L152 (83.2837, 62.6271) -> (81.9375, 62.6271)
  line L153 (81.9375, 62.6271) -> (81.9375, 62.9254)
  line L154 (81.9375, 62.9254) -> (83.4134, 65.0291)
  line L155 (83.4134, 65.0291) -> (83.6702, 65.0291)
  line L156 (83.6702, 65.0291) -> (83.6702, 62.9591)
  line L157 (83.6702, 62.9591) -> (84.0956, 62.9591)
  line L158 (83.2837, 62.9591) -> (83.2837, 64.5363)
  line L159 (83.2837, 64.5363) -> (82.1683, 62.9591)
  line L160 (82.1683, 62.9591) -> (83.2837, 62.9591)
  line L161 (86.3446, 64.9643) -> (86.163, 64.5674)
  line L162 (86.163, 64.5674) -> (85.2085, 64.5674)
  line L163 (85.2085, 64.5674) -> (84.9983, 64.142)
  spline S269 degree 2 poles (84.9983, 64.142) (85.6183, 64.0512) (85.9815, 63.6803) knots 0 0 0 1 1 1
  spline S270 degree 2 poles (85.9815, 63.6803) (86.2927, 63.3612) (86.2927, 62.9306) knots 0 0 0 1 1 1
  spline S271 degree 2 poles (86.2927, 62.9306) (86.2927, 62.6816) (86.0878, 62.2536) (85.7791, 61.9553) (85.5898, 61.8645) knots 0 0 0 1 2 3 3 3
  spline S272 degree 2 poles (85.5898, 61.8645) (85.32, 61.7348) (85.0373, 61.7348) knots 0 0 0 1 1 1
  spline S273 degree 2 poles (85.0373, 61.7348) (84.7493, 61.7348) (84.4899, 61.9293) (84.4899, 62.0461) knots 0 0 0 1 2 2 2
  spline S274 degree 2 poles (84.4899, 62.0461) (84.4899, 62.1109) (84.5963, 62.2121) (84.6793, 62.2121) knots 0 0 0 1 2 2 2
  spline S275 degree 2 poles (84.6793, 62.2121) (84.7389, 62.2121) (84.8323, 62.1732) (84.9413, 62.0954) knots 0 0 0 1 2 2 2
  spline S276 degree 2 poles (84.9413, 62.0954) (85.1177, 61.976) (85.2992, 61.9734) knots 0 0 0 1 1 1
  spline S277 degree 2 poles (85.2992, 61.9734) (85.5716, 61.9734) (85.9892, 62.3885) (85.9892, 62.6868) knots 0 0 0 1 2 2 2
  spline S278 degree 2 poles (85.9892, 62.6868) (85.9892, 62.9747) (85.6183, 63.4753) (85.2915, 63.6102) knots 0 0 0 1 2 2 2
  spline S279 degree 2 poles (85.2915, 63.6102) (85.0373, 63.7166) (84.5963, 63.7321) knots 0 0 0 1 1 1
  line L164 (84.5963, 63.7321) -> (85.2059, 64.9643)
  line L165 (85.2059, 64.9643) -> (86.3446, 64.9643)
  line L166 (50.5493, 57.8285) -> (49.3146, 57.8285)
  line L167 (49.3146, 57.8285) -> (49.0993, 57.3304)
  spline S280 degree 2 poles (49.0993, 57.3304) (49.0189, 57.1437) (49.0189, 57.0529) knots 0 0 0 1 1 1
  spline S281 degree 2 poles (49.0189, 57.0529) (49.0189, 56.9803) (49.159, 56.8687) (49.3872, 56.8532) knots 0 0 0 1 2 2 2
  line L168 (49.3872, 56.8532) -> (49.3872, 56.7676)
  line L169 (49.3872, 56.7676) -> (48.386, 56.7676)
  line L170 (48.386, 56.7676) -> (48.386, 56.8532)
  spline S282 degree 2 poles (48.386, 56.8532) (48.5857, 56.8895) (48.6428, 56.9439) knots 0 0 0 1 1 1
  spline S283 degree 2 poles (48.6428, 56.9439) (48.7621, 57.0581) (48.9074, 57.4031) knots 0 0 0 1 1 1
  line L171 (48.9074, 57.4031) -> (50.0279, 60.0152)
  line L172 (50.0279, 60.0152) -> (50.111, 60.0152)
  line L173 (50.111, 60.0152) -> (51.216, 57.3745)
  spline S284 degree 2 poles (51.216, 57.3745) (51.3483, 57.0555) (51.5662, 56.8661) (51.7607, 56.8532) knots 0 0 0 1 2 2 2
  line L174 (51.7607, 56.8532) -> (51.7607, 56.7676)
  line L175 (51.7607, 56.7676) -> (50.5078, 56.7676)
  line L176 (50.5078, 56.7676) -> (50.5078, 56.8532)
  spline S285 degree 2 poles (50.5078, 56.8532) (50.6972, 56.8635) (50.8321, 56.9699) (50.8321, 57.0477) knots 0 0 0 1 2 2 2
  spline S286 degree 2 poles (50.8321, 57.0477) (50.8321, 57.1515) (50.7387, 57.3745) knots 0 0 0 1 1 1
  line L177 (50.7387, 57.3745) -> (50.5493, 57.8285)
  line L178 (50.4767, 58.0023) -> (49.9423, 59.2863)
  line L179 (49.9423, 59.2863) -> (49.3872, 58.0023)
  line L180 (49.3872, 58.0023) -> (50.4767, 58.0023)
  line L181 (53.8437, 58.9128) -> (53.8437, 57.6106)
  spline S287 degree 2 poles (53.8437, 57.6106) (53.8437, 57.2423) (53.88, 57.0762) (53.9552, 57.0114) (54.0071, 57.0114) knots 0 0 0 1 2 3 3 3
  spline S288 degree 2 poles (54.0071, 57.0114) (54.0797, 57.0114) (54.1705, 57.0503) knots 0 0 0 1 1 1
  line L182 (54.1705, 57.0503) -> (54.2042, 56.9647)
  line L183 (54.2042, 56.9647) -> (53.5635, 56.7027)
  line L184 (53.5635, 56.7027) -> (53.4572, 56.7027)
  line L185 (53.4572, 56.7027) -> (53.4572, 57.1567)
  spline S289 degree 2 poles (53.4572, 57.1567) (53.1796, 56.8583) (52.8917, 56.7027) (52.7283, 56.7027) knots 0 0 0 1 2 2 2
  spline S290 degree 2 poles (52.7283, 56.7027) (52.5493, 56.7027) (52.2847, 56.9102) (52.1809, 57.2397) (52.1809, 57.538) knots 0 0 0 1 2 3 3 3
  line L186 (52.1809, 57.538) -> (52.1809, 58.4951)
  spline S291 degree 2 poles (52.1809, 58.4951) (52.1809, 58.6482) (52.1161, 58.7649) (51.9864, 58.8298) (51.8178, 58.8272) knots 0 0 0 1 2 3 3 3
  line L187 (51.8178, 58.8272) -> (51.8178, 58.9128)
  line L188 (51.8178, 58.9128) -> (52.57, 58.9128)
  line L189 (52.57, 58.9128) -> (52.57, 57.4783)
  spline S292 degree 2 poles (52.57, 57.4783) (52.57, 57.1774) (52.7775, 56.9906) (52.9254, 56.9906) knots 0 0 0 1 2 2 2
  spline S293 degree 2 poles (52.9254, 56.9906) (53.0266, 56.9906) (53.2808, 57.1177) (53.4572, 57.2941) knots 0 0 0 1 2 2 2
  line L190 (53.4572, 57.2941) -> (53.4572, 58.5107)
  spline S294 degree 2 poles (53.4572, 58.5107) (53.4572, 58.6923) (53.3223, 58.822) (53.1096, 58.8272) knots 0 0 0 1 2 2 2
  line L191 (53.1096, 58.8272) -> (53.1096, 58.9128)
  line L192 (53.1096, 58.9128) -> (53.8437, 58.9128)
  spline S295 degree 2 poles (54.9357, 57.5509) (54.7386, 57.6469) (54.5285, 57.9893) (54.5285, 58.1994) knots 0 0 0 1 2 2 2
  spline S296 degree 2 poles (54.5285, 58.1994) (54.5285, 58.5159) (55.0083, 58.975) (55.3845, 58.975) knots 0 0 0 1 2 2 2
  spline S297 degree 2 poles (55.3845, 58.975) (55.6906, 58.975) (55.9162, 58.8246) knots 0 0 0 1 1 1
  line L193 (55.9162, 58.8246) -> (56.3702, 58.8246)
  spline S298 degree 2 poles (56.3702, 58.8246) (56.4713, 58.8246) (56.5051, 58.8142) (56.5128, 58.7986) knots 0 0 0 1 2 2 2
  spline S299 degree 2 poles (56.5128, 58.7986) (56.5258, 58.7779) (56.5258, 58.7234) knots 0 0 0 1 1 1
  spline S300 degree 2 poles (56.5258, 58.7234) (56.5258, 58.6637) (56.5128, 58.6404) knots 0 0 0 1 1 1
  spline S301 degree 2 poles (56.5128, 58.6404) (56.5076, 58.6274) (56.4713, 58.6145) (56.3702, 58.6145) knots 0 0 0 1 2 2 2
  line L194 (56.3702, 58.6145) -> (56.09, 58.6145)
  spline S302 degree 2 poles (56.09, 58.6145) (56.2223, 58.4458) (56.2223, 58.1839) knots 0 0 0 1 1 1
  spline S303 degree 2 poles (56.2223, 58.1839) (56.2223, 57.883) (55.7632, 57.4575) (55.3767, 57.4575) knots 0 0 0 1 2 2 2
  spline S304 degree 2 poles (55.3767, 57.4575) (55.2185, 57.4575) (55.0498, 57.5042) knots 0 0 0 1 1 1
  spline S305 degree 2 poles (55.0498, 57.5042) (54.9487, 57.416) (54.876, 57.2838) (54.876, 57.2371) knots 0 0 0 1 2 2 2
  spline S306 degree 2 poles (54.876, 57.2371) (54.876, 57.1956) (54.9539, 57.1203) (55.0654, 57.1048) knots 0 0 0 1 2 2 2
  spline S307 degree 2 poles (55.0654, 57.1048) (55.1303, 57.0944) (55.3948, 57.0892) knots 0 0 0 1 1 1
  spline S308 degree 2 poles (55.3948, 57.0892) (55.8773, 57.0762) (56.02, 57.0555) knots 0 0 0 1 1 1
  spline S309 degree 2 poles (56.02, 57.0555) (56.2379, 57.0244) (56.4973, 56.7624) (56.4973, 56.573) knots 0 0 0 1 2 2 2
  spline S310 degree 2 poles (56.4973, 56.573) (56.4973, 56.3084) (56.2483, 56.0776) knots 0 0 0 1 1 1
  spline S311 degree 2 poles (56.2483, 56.0776) (55.8825, 55.7352) (55.2937, 55.7352) knots 0 0 0 1 1 1
  spline S312 degree 2 poles (55.2937, 55.7352) (54.8423, 55.7352) (54.5311, 55.9375) knots 0 0 0 1 1 1
  spline S313 degree 2 poles (54.5311, 55.9375) (54.3547, 56.0542) (54.3547, 56.1813) knots 0 0 0 1 1 1
  spline S314 degree 2 poles (54.3547, 56.1813) (54.3547, 56.2384) (54.3806, 56.2929) knots 0 0 0 1 1 1
  spline S315 degree 2 poles (54.3806, 56.2929) (54.4195, 56.3811) (54.544, 56.5341) knots 0 0 0 1 1 1